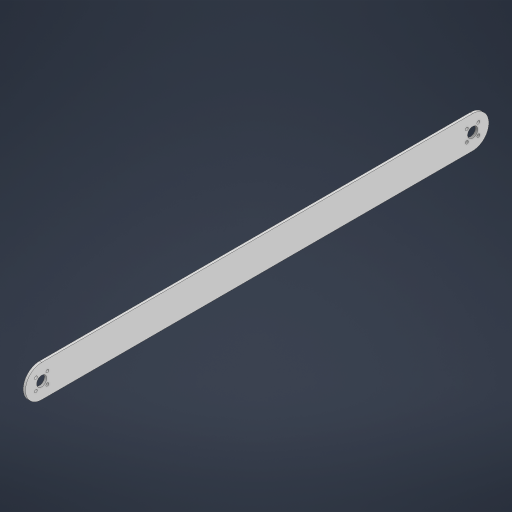
# Autodesk Inventor part: ArmBarStage1
Saved by Autodesk Inventor 2024 (Build 280153000, 153)
## iProperties
Created: 2023-10-20
Part Number: ArmBarStage1
Material: Generic
Document SubType Name: Modeling
Designer: avsar
Density: 1 g/cm^3
Appearance: Default
Author: avsar
Autodesk Inventor part; units mm, degrees
ref_plane "YZ Plane" through (0, 0, 0) normal (1, 0, 0) x (0, 1, 0)
ref_plane "XZ Plane" through (0, 0, 0) normal (0, 1, 0) x (-1, 0, 0)
ref_plane "XY Plane" through (0, 0, 0) normal (0, 0, 1) x (1, 0, 0)
sketch "Sketch1" plane through (0, 0, 0) normal (1, 0, 0) x (0, 1, 0)
  line L0 (-22.5, 300) -> (22.5, 300) construction
  line L1 (22.5, 300) -> (22.5, -300)
  line L2 (22.5, -300) -> (-22.5, -300) construction
  line L3 (-22.5, -300) -> (-22.5, 300)
  line L4 (-22.5, 300) -> (22.5, -300) construction
  line L5 (22.5, 300) -> (-22.5, -300) construction
  arc A0 (-22.5, -300) -> (22.5, -300) centre (0, -300) ccw
  arc A1 (22.5, 300) -> (-22.5, 300) centre (0, 300) ccw
  point P0 (0, 0)
  dimension "d0" = 45
  dimension "d1" = 600
  constraints: 12 end point, 4 point on circle, 3 tangent, 2 centre point, 2 midpoint, 2 parallel, 1 horizontal, 1 perpendicular
  measures "d0" distance of L1.end L2.end
  measures "d1" distance of L0.end L1.end
extrude "Extrusion2" add sketch "Sketch1" along normal mid plane 3.175
sketch "Sketch3" plane through (1.5875, 0, 0) normal (1, 0, 0) x (0, 0, -1)
  line L0 (300, 22.5) -> (-300, 22.5) construction
  arc A0 (-300, 22.5) -> (-300, -22.5) centre (-300, 0) ccw construction
  line L1 (-300, -22.5) -> (300, -22.5) construction
  arc A1 (300, -22.5) -> (300, 22.5) centre (300, 0) ccw construction
  circle A2 centre (-300, 0) radius 7
  circle A3 centre (-308, 8) radius 2
  circle A4 centre (-308, -8) radius 2
  circle A5 centre (-292, -8) radius 2
  circle A6 centre (-292, 8) radius 2
  line L2 (0, 22.5) -> (0, -22.5) construction
  circle A7 centre (300, 0) radius 7
  circle A8 centre (308, 8) radius 2
  circle A9 centre (308, -8) radius 2
  circle A10 centre (292, -8) radius 2
  circle A11 centre (292, 8) radius 2
  point P0 (0, 0)
  dimension "d14" = 14
  dimension "d15" = 4
  dimension "d16" = 8
  dimension "d17" = 8
  dimension "d20" = 360
  constraints: 10 centre point, 6 symmetric about line, 2 coincident, 2 end point, 2 midpoint, 14 other
  measures "d14" diameter of A2
  measures "d15" diameter of A3
  measures "d16" horizontal distance of A0.centre A3.centre
  measures "d17" horizontal distance of A0.centre A3.centre
extrude "Extrusion3" cut sketch "Sketch3" against normal through all
body "Solid2"
